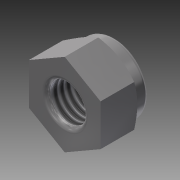
# Autodesk Inventor part: Nylon_Nat(M4)
Saved by Autodesk Inventor 2013 (Build 170138000, 138)
## iProperties
Created: 2013-02-09
Material: ステンレス鋼
Document SubType Name: Modeling
Designer: andou
Density: 8.08 g/cm^3
Mass: 1.63168 g
Surface Area: 2.81381 cm^2
Volume: 0.20194 cm^3
Description: 市販品
Author: andou
Title: Nylon_Nat(M4)
Autodesk Inventor part; units mm, degrees
ref_plane "YZ Plane" through (0, 0, 0) normal (1, 0, 0) x (0, 1, 0)
ref_plane "XZ Plane" through (0, 0, 0) normal (0, 1, 0) x (-1, 0, 0)
ref_plane "XY Plane" through (0, 0, 0) normal (0, 0, 1) x (1, 0, 0)
sketch "スケッチ1" plane through (0, 0, 0) normal (0, 0, 1) x (1, 0, 0)
  line L0 (4.5, 0.9036) -> (4.5, -2.75)
  line L1 (4.5, -2.75) -> (2, -2.75)
  line L2 (0, 2.75) -> (0, -2.75)
  line L3 (3.9, 1.25) -> (4.5, 0.9036)
  line L4 (2, -2.75) -> (2, 2.75)
  line L5 (2, 2.75) -> (3.7, 2.75)
  line L6 (3.9, 1.25) -> (3.7, 1.25)
  line L7 (3.7, 1.25) -> (3.7, 2.75)
  point P0 (0, 0)
  dimension "d3" = 4.5
  dimension "d14" = 2.75
  dimension "d15" = 5.5
  dimension "d16" = 2.75
  dimension "d17" = 5.5
  dimension "d18" = 2.5
  dimension "d20" = 120
  dimension "d28" = 1.7
  dimension "d29" = 1.5
  dimension "d30" = 0.2
  constraints: 16 end point, 2 parallel, 2 perpendicular, 1 horizontal
  measures "d3" distance from line of point (0, 0) L0
  measures "d14" distance from line of point (0, 0) L1
  measures "d15" distance of L2.start L2.end
  measures "d16" distance of L2.end point (0, 0)
  measures "d17" distance between parallel lines of L5 L1
  measures "d18" distance of L0.end L1.end
  measures "d20" angle of L0 L3
  measures "d28" distance of L4.end L5.end
  measures "d29" distance of L6.end L5.end
  measures "d30" distance of L3.start L6.end
revolve "回転1" add sketch "スケッチ1" angle 360 about axis through (0, 2.75, 0) along (0, -1, 0)
sketch "スケッチ3" plane through (0, -2.75, 0) normal (0, -1, 0) x (1, 0, 0)
  circle A0 centre (0, 0) radius 2 projected
  circle A1 centre (0, 0) radius 4.5 projected
  line L0 (0, 4.5) -> (3.8971, 2.25)
  line L1 (3.8971, 2.25) -> (3.8971, -2.25)
  line L2 (3.8971, -2.25) -> (0, -4.5)
  line L3 (0, -4.5) -> (-3.8971, -2.25)
  line L4 (-3.8971, -2.25) -> (-3.8971, 2.25)
  line L5 (-3.8971, 2.25) -> (0, 4.5)
  dimension "d23" = 2.25
  constraints: 12 end point, 1 coincident, 15 other
  measures "d23" vertical distance of L0.end point (0, 0)
extrude "押し出し2" cut sketch "スケッチ3" against normal blind 5.5 contours L1 L2 L3 L4 L5 L0 keep common part
fillet "フィレット1" radius 0.5 2 edges at (-3.7, 2.75, 0) (-2, -2.75, 0)
sketch "スケッチ4" plane through (0, 2.75, 0) normal (0, 1, 0) x (1, 0, 0)
  circle A0 centre (0, 0) radius 2 projected
  circle A1 centre (0, 0) radius 3.2 projected
  circle A2 centre (0, 0) radius 2.5
  dimension "d32" = 5
  constraints: 1 centre point, 1 coincident
  measures "d32" diameter of A2
extrude "押し出し3" cut sketch "スケッチ4" against normal blind 0.2 contours A2
fillet "フィレット2" radius 0.1 2 edges at (-2, 2.55, 0) (-2.5, 2.75, 0)
thread "ねじ3" size "M4x0.7" class "6H" standard "ANSI Metric M Profile" full length
